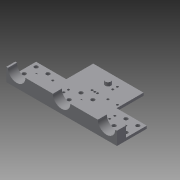
# Autodesk Inventor part: bnc-mount
Saved by Autodesk Inventor 2015 SP1 (Build 190203100, 203)
## iProperties
Created: 2015-03-30
Part Number: bnc-mount
Material: Generic
Document SubType Name: Modeling
Designer: kam42
Density: 1 g/cm^3
Appearance: Default
Author: kam42
Autodesk Inventor part; units mm, degrees
ref_plane "YZ Plane" through (0, 0, 0) normal (1, 0, 0) x (0, 1, 0)
ref_plane "XZ Plane" through (0, 0, 0) normal (0, 1, 0) x (-1, 0, 0)
ref_plane "XY Plane" through (0, 0, 0) normal (0, 0, 1) x (1, 0, 0)
sketch "Sketch1" plane through (0, 0, 0) normal (0, 0, 1) x (1, 0, 0)
  circle A0 centre (0, -0.0241) radius 0.585
  line L0 (-3.3, -3.3241) -> (3.3, -3.3241) construction
  line L1 (3.3, -3.3241) -> (3.3, 3.2759) construction
  line L2 (3.3, 3.2759) -> (-3.3, 3.2759) construction
  line L3 (-3.3, 3.2759) -> (-3.3, -3.3241) construction
  line L4 (-3.3, -3.3241) -> (3.3, 3.2759) construction
  line L5 (3.3, -3.3241) -> (-3.3, 3.2759) construction
  circle A1 centre (-3.3, 3.2759) radius 1.055
  circle A2 centre (3.3, 3.2759) radius 1.055
  circle A3 centre (-3.3, -3.3241) radius 1.055
  circle A4 centre (3.3, -3.3241) radius 1.055
  circle A5 centre (25, -0.0241) radius 0.585
  circle A6 centre (21.7, 3.2759) radius 1.055
  circle A7 centre (28.3, 3.2759) radius 1.055
  circle A8 centre (21.7, -3.3241) radius 1.055
  circle A9 centre (28.3, -3.3241) radius 1.055
  circle A10 centre (50, -0.0241) radius 0.585
  circle A11 centre (46.7, 3.2759) radius 1.055
  circle A12 centre (53.3, 3.2759) radius 1.055
  circle A13 centre (46.7, -3.3241) radius 1.055
  circle A14 centre (53.3, -3.3241) radius 1.055
  line L6 (-5.8, 5.7759) -> (55.8, 5.7759)
  line L7 (55.8, 5.7759) -> (55.8, -10.8241)
  line L8 (55.8, -10.8241) -> (-5.8, -10.8241)
  line L9 (-5.8, -10.8241) -> (-5.8, 5.7759)
  line L10 (-0.4, 5.7759) -> (50.4, 5.7759)
  line L11 (50.4, 5.7759) -> (50.4, 20.7759)
  line L12 (50.4, 20.7759) -> (-0.4, 20.7759)
  line L13 (-0.4, 20.7759) -> (-0.4, 5.7759)
  line L14 (-0.4, 20.7759) -> (50.4, 5.7759) construction
  line L15 (50.4, 20.7759) -> (-0.4, 5.7759) construction
  circle A15 centre (2.85, 9.7759) radius 1.6472
  circle A16 centre (47.15, 9.7759) radius 1.4098
  point P0 (25, 13.2759)
  dimension "d6" = 6.6
  dimension "d7" = 6.6
  dimension "d8" = 1.17
  dimension "d9" = 2.11
  dimension "d10" = 2.11
  dimension "d11" = 2.11
  dimension "d12" = 2.11
  dimension "d15" = 25
  dimension "d21" = 2.5
  dimension "d22" = 2.5
  dimension "d23" = 2.5
  dimension "d24" = 7.5
  dimension "d27" = 50.8
  dimension "d28" = 15
  dimension "d29" = 44.3
  dimension "d30" = 22.15
  dimension "d31" = 4
  constraints: 32 end point, 17 centre point, 6 parallel, 4 coincident, 4 horizontal, 3 midpoint, 3 perpendicular, 1 horizontal alignment, 1 point on line, 20 other
  measures "d6" distance of L0.end L1.end
  measures "d7" distance of L1.end L2.end
  measures "d8" diameter of A0
  measures "d9" diameter of A1
  measures "d10" diameter of A2
  measures "d11" diameter of A4
  measures "d12" diameter of A3
  measures "d15" distance of A2.centre A7.centre
  measures "d21" distance from line of L7 A12.centre
  measures "d22" distance from line of L9 L2.end
  measures "d23" distance from line of L6 A1.centre
  measures "d24" distance from line of L8 L0.start
  measures "d27" distance of L11.end L12.end
  measures "d28" distance of L12.end L10.start
  measures "d29" distance of A16.centre A15.centre
  measures "d30" horizontal distance of point (25, 13.276) A15.centre
  measures "d31" distance from line of A15.centre L10
extrude "Extrusion1" add sketch "Sketch1" along normal blind 1.5
sketch "Sketch3" plane through (-5.8, -10.8241, 0) normal (0, -1, 0) x (1, 0, 0)
  line L0 (0, 1.5) -> (61.6, 1.5) projected
  line L1 (6.385, 0) -> (6.385, 1.5) projected
  line L2 (5.215, 0) -> (5.215, 1.5) projected
  line L3 (30.215, 0) -> (30.215, 1.5) projected
  line L4 (31.385, 0) -> (31.385, 1.5) projected
  line L5 (55.215, 0) -> (55.215, 1.5) projected
  line L6 (56.385, 0) -> (56.385, 1.5) projected
  arc A0 (0.95, 7.35) -> (10.65, 7.35) centre (5.8, 7.35) ccw
  arc A1 (25.95, 7.35) -> (35.65, 7.35) centre (30.8, 7.35) ccw
  arc A2 (50.95, 7.35) -> (60.65, 7.35) centre (55.8, 7.35) ccw
  line L7 (0, 1.5) -> (61.6, 1.5)
  line L8 (61.6, 1.5) -> (61.6, 7.35)
  line L9 (0, 7.35) -> (0, 1.5)
  line L10 (61.6, 7.35) -> (60.65, 7.35)
  line L11 (50.95, 7.35) -> (35.65, 7.35)
  line L12 (25.95, 7.35) -> (10.65, 7.35)
  line L13 (0.95, 7.35) -> (0, 7.35)
  point P0 (5.8, 0)
  dimension "d36" = 9.7
  dimension "d37" = 9.7
  dimension "d38" = 5.85
  dimension "d39" = 9.7
  dimension "d40" = 0.585
  constraints: 14 end point, 6 point on circle, 5 parallel, 3 centre point, 2 horizontal alignment, 1 horizontal, 1 perpendicular
  measures "d36" diameter of A0
  measures "d37" diameter of A1
  measures "d38" distance from line of A0.centre L0
  measures "d39" diameter of A2
  measures "d40" distance from line of A2.centre L5
extrude "Extrusion2" add sketch "Sketch3" against normal blind 5
sketch "Sketch4" plane through (0, 0, 1.5) normal (0, 0, 1) x (1, 0, 0)
  circle A0 centre (2.85, 9.7759) radius 1.6472 projected
  circle A1 centre (47.15, 9.7759) radius 1.4098 projected
  point P0 (0, 0)
  point P1 (16.6938, 1.3126)
  point P2 (16.6938, -1.2274)
  point P3 (42.15, 1.6758)
  point P4 (42.15, -1.2274)
  point P5 (7.85, 1.4313)
  point P6 (7.85, -1.0281)
  point P7 (25, 7.6611)
  point P8 (26.5, 7.6611)
  point P9 (23.5, 7.6611)
  point P10 (32.315, 7.6611)
  point P11 (37.565, 7.6611)
  dimension "d43" = 2.54
  dimension "d44" = 5
  dimension "d45" = 5
  dimension "d56" = 1.5
  dimension "d57" = 1.5
  dimension "d72" = 5.25
  constraints: 3 vertical alignment, 2 horizontal alignment
  measures "d43" distance of point (16.694, -1.227) point (16.694, 1.313)
  measures "d44" horizontal distance of point (7.85, -1.028) A0.centre
  measures "d45" horizontal distance of A1.centre point (42.15, 1.676)
  measures "d56" distance of point (26.5, 7.661) point (25, 7.661)
  measures "d57" distance of point (25, 7.661) point (23.5, 7.661)
  measures "d72" distance of point (37.565, 7.661) point (32.315, 7.661)
hole "Hole1" at (7.85, 1.4313, 1.5) at (7.85, -1.0281, 1.5) at (16.6938, 1.3126, 1.5) at (16.6938, -1.2274, 1.5) at (42.15, 1.6758, 1.5) at (42.15, -1.2274, 1.5) at (23.5, 7.6611, 1.5) at (25, 7.6611, 1.5) at (26.5, 7.6611, 1.5) at (37.565, 7.6611, 1.5) at (32.315, 7.6611, 1.5) direction (0, 0, -1) diameter 1.25 end through all
sketch "Sketch7" plane through (0, 0, 1.5) normal (0, 0, 1) x (1, 0, 0)
  circle A0 centre (25, 15.0281) radius 1.6
  point P0 (0, 0)
  dimension "d61" = 3.2
  constraints: 1 centre point
  measures "d61" diameter of A0
extrude "Extrusion3" add sketch "Sketch7" along normal blind 2
sketch "Sketch8" plane through (0, 0, 1.5) normal (0, 0, 1) x (1, 0, 0)
  point P0 (0, 0)
  point P1 (28.8706, 16.3411)
  point P2 (28.8706, 13.8011)
  dimension "d64" = 2.54
  constraints: 1 vertical alignment
  measures "d64" distance of point (28.871, 13.801) point (28.871, 16.341)
hole "Hole2" at (28.8706, 16.3411, 1.5) at (28.8706, 13.8011, 1.5) direction (0, 0, -1) diameter 1.25 end through all
sketch "Sketch9" plane through (0, 0, 1.5) normal (0, 0, 1) x (1, 0, 0)
  circle A0 centre (25, 15.0281) radius 1.6 projected
  line L0 (50.4, 20.7759) -> (-0.4, 20.7759) projected
  circle A1 centre (2.85, 9.7759) radius 1.6472 projected
  circle A2 centre (47.15, 9.7759) radius 1.4098 projected
  line L1 (39, 9.2804) -> (11, 9.2804)
  line L2 (11, 9.2804) -> (11, 20.7759)
  line L3 (11, 20.7759) -> (39, 20.7759)
  line L4 (39, 20.7759) -> (39, 9.2804)
  line L5 (39, 9.2804) -> (11, 20.7759) construction
  line L6 (11, 9.2804) -> (39, 20.7759) construction
  line L7 (-0.4, 5.7759) -> (11, 5.7759)
  line L8 (11, 5.7759) -> (11, 20.7759)
  line L9 (11, 20.7759) -> (-0.4, 20.7759)
  line L10 (-0.4, 20.7759) -> (-0.4, 5.7759)
  line L11 (50.4, 5.7759) -> (39, 5.7759)
  line L12 (39, 5.7759) -> (39, 20.7759)
  line L13 (39, 20.7759) -> (50.4, 20.7759)
  line L14 (50.4, 20.7759) -> (50.4, 5.7759)
  point P0 (0, 0)
  dimension "d74" = 28
  constraints: 28 end point, 6 parallel, 3 horizontal, 3 perpendicular, 2 midpoint, 1 point on line
  measures "d74" distance of L2.end L3.end
extrude "Extrusion4" cut sketch "Sketch9" against normal up to next contours L14 L11 L12 L4 L0 | L2 L8 L7 L10 L0
body "Solid1"
